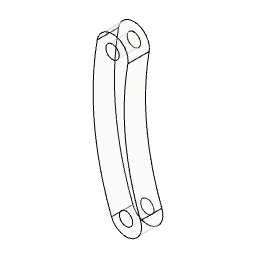
AssemblyThrowerRamp v2 (Autodesk Fusion 360 archive; units mm, degrees)
design "RampSeparator"
Autodesk Fusion 360 part; units mm, degrees
sketch "Sketch1" plane through (0, 0, 0) normal (0, 1, 0) x (1, 0, 0)
  circle A0 centre (0, 0) radius 14 construction
  line L0 (0, 0) -> (0, 52) construction
  circle A1 centre (0, 0) radius 58 construction
  line L1 (0, 0) -> (-58, 0) construction
  line L2 (-61.5, 0) -> (-54.5, 0) construction
  line L3 (-52.0547, 32.75) -> (-43.5625, 32.75) construction
  line L4 (-54.7818, 27.95) -> (-46.7873, 27.95) construction
  line L5 (-59.0893, -17.05) -> (-51.7643, -17.05) construction
  circle A2 centre (-57.1227, -10.05) radius 1.5
  circle A3 centre (-54.0842, 20.95) radius 1.5
  arc A4 (-50.8205, 19.6858) -> (-57.3479, 22.2142) centre (-54.0842, 20.95) ccw
  arc A5 (-57.3479, 22.2142) -> (-55.2493, 17.6496) centre (-54.0842, 20.95) ccw construction
  arc A6 (-55.2493, 17.6496) -> (-50.8205, 19.6858) centre (-54.0842, 20.95) ccw construction
  arc A7 (-60.5697, -10.6565) -> (-53.6756, -9.4435) centre (-57.1227, -10.05) ccw
  arc A8 (-57.6248, -6.5862) -> (-60.5697, -10.6565) centre (-57.1227, -10.05) ccw construction
  arc A9 (-53.6756, -9.4435) -> (-57.6248, -6.5862) centre (-57.1227, -10.05) ccw construction
  arc A10 (-60.5697, -10.6565) -> (-59.0893, -17.05) centre (0, 0) ccw construction
  arc A11 (-53.6756, -9.4435) -> (-51.7643, -17.05) centre (0, 0) ccw construction
  arc A12 (-51.7643, -17.05) -> (-46.7873, 27.95) centre (0, 0) ccw construction
  arc A13 (-50.8205, 19.6858) -> (-53.6756, -9.4435) centre (0, 0) ccw
  arc A14 (-46.7873, 27.95) -> (-50.8205, 19.6858) centre (0, 0) ccw construction
  arc A15 (-59.0893, -17.05) -> (-54.7818, 27.95) centre (0, 0) ccw construction
  arc A16 (-57.3479, 22.2142) -> (-60.5697, -10.6565) centre (0, 0) ccw
  arc A17 (-54.7818, 27.95) -> (-57.3479, 22.2142) centre (0, 0) ccw construction
  point P0 (0, 14)
  point P1 (-58, 0)
  point P2 (-54.0842, 20.95)
  point P3 (-57.1227, -10.05)
  dimension "d6" = 28
  dimension "d7" = 38
  dimension "d8" = 116
  dimension "d9" = 7
  dimension "d10" = 19.25
  dimension "d11" = 4.8
  dimension "d12" = 7
  dimension "d13" = 45
  dimension "d14" = 7
  dimension "d15" = 3
  dimension "d16" = 3
  constraint coincident A0.centre L0.start
  constraint vertical L0
  constraint coincident A0 P0
  constraint coincident L0 P0
  constraint coincident A1 P1
  constraint perpendicular L0 L1
  constraint perpendicular L0 L2
  constraint midpoint L2 P1
  constraint coincident P1 L1.end
  constraint concentric A0 A12
  constraint coincident L2.end A12
  constraint concentric A12 A15
  constraint coincident L2.start A15
  constraint coincident L3.start A15
  constraint coincident L3.end A12
  constraint horizontal L3
  constraint horizontal L4
  constraint coincident A1 P2
  constraint horizontal L5
  constraint coincident A1 P3
  constraint coincident P3 A2.centre
  constraint coincident P2 A3.centre
  constraint tangent A7 A12
  constraint concentric A3 A4
  constraint tangent A4 A12
  constraint coincident A4.end A15
  constraint coincident A1 A5.end
  constraint concentric A4 A5
  constraint coincident A4.start A12
  constraint concentric A4 A6
  constraint coincident A1 A8.start
  constraint concentric A7 A8
  constraint concentric A7 A9
  constraint concentric A10 A15
  constraint concentric A11 A12
  constraint concentric A12 A13
  constraint concentric A12 A14
  constraint concentric A15 A16
  constraint concentric A15 A17
  measures "d6" diameter of A0
  measures "d7" distance of L0.end P0
  measures "d8" diameter of A1
  measures "d9" distance of L2.start L2.end
  measures "d10" distance of L0.end L3
  measures "d11" distance of L3 L4
  measures "d12" distance of L4 P2
  measures "d13" distance of L4 L5
  measures "d14" distance of L5 P3
  measures "d15" diameter of A2
  measures "d16" diameter of A3
extrude "Extrude1" add sketch "Sketch1" along normal blind 4.8

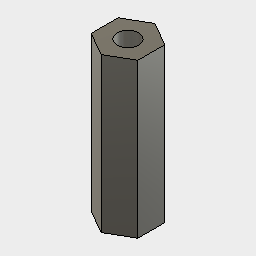
design "Spacer M3x18"
Autodesk Fusion 360 part; units mm, degrees
sketch "Sketch1" plane through (0, 0, 0) normal (0, 1, 0) x (1, 0, 0)
  line L0 (2.725, 1.5733) -> (0, 3.1466)
  line L1 (0, 3.1466) -> (-2.725, 1.5733)
  line L2 (-2.725, 1.5733) -> (-2.725, -1.5733)
  line L3 (-2.725, -1.5733) -> (0, -3.1466)
  line L4 (0, -3.1466) -> (2.725, -1.5733)
  line L5 (2.725, -1.5733) -> (2.725, 1.5733)
  circle A0 centre (0, 0) radius 1.25
  dimension "d1" = 2.5
  measures "d1" diameter of A0
extrude "Extrude1" add sketch "Sketch1" along normal blind 18
